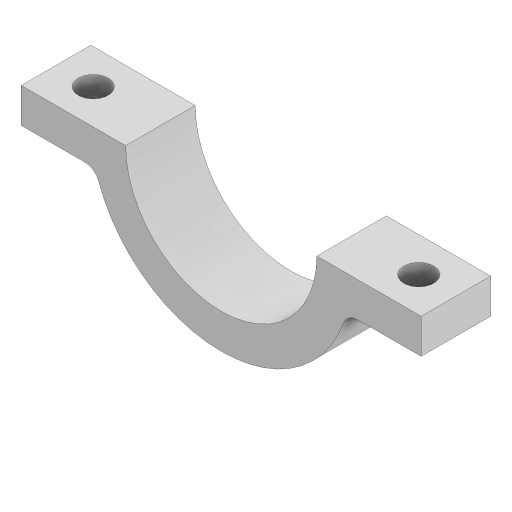
# Autodesk Inventor part: Part1
Saved by Autodesk Inventor 2023.3 (Build 273359000, 359)
## iProperties
Created: 2025-06-02
Part Number: Part1
Material: Generic
Document SubType Name: Modeling
Designer: David Zindović
Density: 1 g/cm^3
Appearance: Default
Author: David Zindović
Autodesk Inventor part; units mm, degrees
ref_plane "YZ Plane" through (0, 0, 0) normal (1, 0, 0) x (0, 1, 0)
ref_plane "XZ Plane" through (0, 0, 0) normal (0, 1, 0) x (-1, 0, 0)
ref_plane "XY Plane" through (0, 0, 0) normal (0, 0, 1) x (1, 0, 0)
sketch "Sketch1" plane through (0, 0, 0) normal (0, 0, 1) x (1, 0, 0)
  circle A0 centre (0, 0) radius 13.75
  circle A1 centre (0, 0) radius 18.75
  line L0 (-18.75, 0) -> (-28.75, 0)
  line L1 (-28.75, 0) -> (-28.75, -5)
  line L2 (-28.75, -5) -> (-18.75, -5)
  line L3 (-18.75, -5) -> (-18.75, 0)
  line L4 (-18.75, -5) -> (-13.75, -5)
  line L5 (-13.75, -5) -> (-13.75, 0)
  line L6 (-13.75, 0) -> (-18.75, 0)
  line L7 (-18.75, 0) -> (-18.75, -5)
  line L8 (18.75, 0) -> (28.75, 0)
  line L9 (28.75, 0) -> (28.75, -5)
  line L10 (28.75, -5) -> (18.75, -5)
  line L11 (18.75, -5) -> (18.75, 0)
  line L12 (18.75, -5) -> (13.75, -5)
  line L13 (13.75, -5) -> (13.75, 0)
  line L14 (13.75, 0) -> (18.75, 0)
  line L15 (18.75, 0) -> (18.75, -5)
  point P0 (-18.071, -5)
  point P1 (18.071, -5)
  dimension "d0" = 27.5
  dimension "d1" = 5
  dimension "d2" = 5
  dimension "d3" = 10
  dimension "d4" = 10
  dimension "d5" = 5
  constraints: 32 end point, 8 parallel, 4 horizontal, 4 perpendicular, 4 point on circle, 2 centre point, 1 coincident, 1 point on line
  measures "d0" diameter of A0
  measures "d1" radial gap between concentric circles of A0 A1
  measures "d2" distance of L1.end L0.end
  measures "d3" distance of L1.end L2.end
  measures "d4" distance of L9.end L10.end
  measures "d5" distance of L8.end L9.end
extrude "Extrusion1" add sketch "Sketch1" along normal blind 10 contours L13 L12 A1 L4 L5 A0 | L14 A1 L12 L13 | L5 L4 A1 L6 | L11 L12 A1 | L8 L9 L10 L11 | L3 L2 L1 L0 | A1 L4 L3
sketch "Sketch2" plane through (-28.75, -5, 0) normal (0, -1, 0) x (1, 0, 0)
  line L0 (0, 0) -> (10.679, 0) projected
  line L1 (10.679, 0) -> (10.679, 10) projected
  line L2 (0, 10) -> (10.679, 10) projected
  line L3 (0, 0) -> (0, 10) projected
  line L4 (46.821, 0) -> (57.5, 0) projected
  line L5 (57.5, 0) -> (57.5, 10) projected
  line L6 (46.821, 10) -> (57.5, 10) projected
  line L7 (46.821, 0) -> (46.821, 10) projected
  circle A0 centre (5.3395, 5) radius 2.15
  circle A1 centre (52.1605, 5) radius 2.15
  point P0 (28.75, 0)
  point P1 (5.3395, 10)
  point P2 (0, 5)
  point P3 (52.1605, 10)
  point P4 (57.5, 5)
  dimension "d8" = 4.3
  dimension "d9" = 4.3
  constraints: 4 midpoint, 2 centre point, 2 horizontal alignment, 2 vertical alignment
  measures "d8" diameter of A0
  measures "d9" diameter of A1
extrude "Extrusion2" cut sketch "Sketch2" against normal up to surface (5 mm away) contours A0 | A1
fillet "Fillet1" radius 2 2 edges at (-18.071, -5, 5) (18.071, -5, 5)
body "Solid1"
